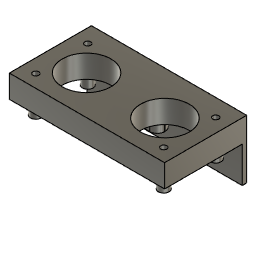
Ultrasonic Sensor Mount (Autodesk Fusion 360 design; units mm, degrees)
Autodesk Fusion 360 part; units mm, degrees
ref_plane "WorkPlane1" through (-22.725, -10, 13.61) normal (0, 0, 1) x (1, 0, 0)
sketch "Sketch1" plane through (0, 0, 13.61) normal (0, 0, 1) x (1, 0, 0)
  circle A0 centre (13.12, 0) radius 8
  circle A1 centre (-13.12, 0) radius 8
  circle A2 centre (-13.12, 0) radius 8.12
  circle A3 centre (13.12, 0) radius 8.12
  line L0 (26, -13) -> (-26, -13)
  line L1 (-26, -13) -> (-26, 13)
  line L2 (-26, 13) -> (26, 13)
  line L3 (26, 13) -> (26, -13)
  line L4 (26, -13) -> (-26, 13) construction
  line L5 (-26, -13) -> (26, 13) construction
  constraint concentric A1 A2
  constraint concentric A0 A3
  constraint horizontal L0
  constraint perpendicular L0 L1
  constraint parallel L0 L2
  constraint parallel L1 L3
  constraint coincident L4 origin
  constraint coincident L5 origin
extrude "Extrude1" add sketch "Sketch1" against normal blind 7.62 contours L0 L1 L2 L3
sketch "Sketch2" plane through (0, 0, 5.99) normal (0, 0, -1) x (-1, 0, 0)
  circle A0 centre (13.12, 0) radius 8.12
  circle A1 centre (-13.12, 0) radius 8.12
  line L0 (26, 13) -> (-26, 13)
  line L1 (-26, 13) -> (-26, -13)
  line L2 (-26, -13) -> (26, -13)
  line L3 (26, -13) -> (26, 13)
  arc A2 (5, 7.4356) -> (3.2, 9.2356) centre (3.2, 7.4356) ccw
  line L4 (5, 7.4356) -> (5, 7.3356)
  arc A3 (3.2, 5.5356) -> (5, 7.3356) centre (3.2, 7.3356) ccw
  line L5 (-3.2, 9.2356) -> (3.2, 9.2356)
  line L6 (3.2, 5.5356) -> (-3.2, 5.5356)
  arc A4 (-5, 7.3356) -> (-3.2, 5.5356) centre (-3.2, 7.3356) ccw
  line L7 (-5, 7.3356) -> (-5, 7.4356)
  arc A5 (-3.2, 9.2356) -> (-5, 7.4356) centre (-3.2, 7.4356) ccw
  line L8 (3.2, 9.2356) -> (-3.2, 9.2356)
  line L9 (3.2, 5.5356) -> (-3.2, 5.5356)
  arc A6 (5, 7.4356) -> (3.2, 9.2356) centre (3.2, 7.4356) ccw
  arc A7 (-3.2, 9.2356) -> (-5, 7.4356) centre (-3.2, 7.4356) ccw
  line L10 (5, 7.4356) -> (5, 7.3356)
  arc A8 (3.2, 5.5356) -> (5, 7.3356) centre (3.2, 7.3356) ccw
  arc A9 (-5, 7.3356) -> (-3.2, 5.5356) centre (-3.2, 7.3356) ccw
  line L11 (-5, 7.4356) -> (-5, 7.3356)
  line L12 (-5.1, 7.4356) -> (-5.1, 7.3356)
  arc A10 (-5.1, 7.3356) -> (-3.2, 5.4356) centre (-3.2, 7.3356) ccw
  line L13 (3.2, 5.4356) -> (-3.2, 5.4356)
  arc A11 (3.2, 5.4356) -> (5.1, 7.3356) centre (3.2, 7.3356) ccw
  line L14 (5.1, 7.4356) -> (5.1, 7.3356)
  arc A12 (5.1, 7.4356) -> (3.2, 9.3356) centre (3.2, 7.4356) ccw
  line L15 (3.2, 9.3356) -> (-3.2, 9.3356)
  arc A13 (-3.2, 9.3356) -> (-5.1, 7.4356) centre (-3.2, 7.4356) ccw
  line L16 (-5.7, 7.4356) -> (-5.7, 7.3356)
  arc A14 (-5.7, 7.3356) -> (-3.2, 4.8356) centre (-3.2, 7.3356) ccw
  line L17 (3.2, 4.8356) -> (-3.2, 4.8356)
  arc A15 (3.2, 4.8356) -> (5.7, 7.3356) centre (3.2, 7.3356) ccw
  line L18 (5.7, 7.4356) -> (5.7, 7.3356)
  arc A16 (5.7, 7.4356) -> (3.2, 9.9356) centre (3.2, 7.4356) ccw
  line L19 (3.2, 9.9356) -> (-3.2, 9.9356)
  arc A17 (-3.2, 9.9356) -> (-5.7, 7.4356) centre (-3.2, 7.4356) ccw
  circle A18 centre (21.425, -8.7) radius 1
  circle A19 centre (-21.425, -8.7) radius 1
  circle A20 centre (-21.425, 8.7) radius 1
  circle A21 centre (21.425, 8.7) radius 1
  circle A22 centre (-21.425, -8.7) radius 1.8
  circle A23 centre (-21.425, 8.7) radius 1.8
  circle A24 centre (21.425, 8.7) radius 1.8
  circle A25 centre (21.425, -8.7) radius 1.8
  point P0 (0, 7.3856)
  point P1 (0, 7.3856)
  dimension "d130" = 0.1
  dimension "d131" = 0.7
  dimension "d8" = 3.6
  dimension "d9" = 3.6
  dimension "d10" = 3.6
  dimension "d11" = 3.6
  dimension "d14" = 2
  dimension "d15" = 2
  dimension "d16" = 2
  dimension "d17" = 2
  constraint concentric A2 A6
  constraint concentric A5 A7
  constraint coincident A2.end L5.end
  constraint coincident L5.start A5.start
  constraint coincident A3.start L6.start
  constraint coincident L6.end A4.end
  constraint coincident A2.start L4.start
  constraint coincident L4.end A3.end
  constraint tangent L6 A8
  constraint tangent L4 A8
  constraint tangent L6 A9
  constraint tangent L7 A9
  constraint coincident L7.end A5.end
  constraint tangent A4 L11
  constraint coincident P1 P0
  constraint concentric A20 A23
  constraint concentric A21 A24
  constraint concentric A18 A25
  measures "d130" distance of L11
  measures "d8" diameter of A22
  measures "d9" diameter of A23
  measures "d10" diameter of A24
  measures "d11" diameter of A25
  measures "d14" diameter of A20
  measures "d15" diameter of A21
  measures "d16" diameter of A18
  measures "d17" diameter of A19
extrude "Extrude2" add sketch "Sketch2" along normal blind 3.69 contours L16 A14 L17 A15 L18 A16 L19 A17
sketch "Sketch3" plane through (0, 0, 5.99) normal (0, 0, -1) x (-1, 0, 0)
extrude "Extrude4" cut sketch "Sketch2" against normal through all contours A18 | A19 | A20 | A21
extrude "Extrude6" add sketch "Sketch2" along normal blind 4.38 contours A22 | A23 | A24 | A25
sketch "Sketch4" plane through (0, 13, 0) normal (0, 1, 0) x (-1, 0, 0)
  line L0 (26, 13.61) -> (-26, 13.61)
  line L1 (-26, 13.61) -> (-26, 5.99)
  line L2 (-26, 5.99) -> (26, 5.99)
  line L3 (26, 5.99) -> (26, 13.61)
  line L4 (26, -6.01) -> (-26, -6.01)
  line L5 (-26, -6.01) -> (-26, 25.61)
  line L6 (-26, 25.61) -> (26, 25.61)
  line L7 (26, 25.61) -> (26, -6.01)
  line L8 (5, 5.99) -> (21.24, 5.99)
  dimension "d18" = 12
  dimension "d19" = 12
  constraint horizontal L4
  constraint vertical L5
  constraint horizontal L6
  constraint vertical L7
  measures "d18" distance of L4 L8
  measures "d19" distance of L0 L6
extrude "Extrude7" add sketch "Sketch4" along normal blind 1.5
extrude "Extrude8" cut 1 faces at (8.6667, 13.5, 25.61) along direction (0, 0, -1) up to surface (12 mm away)
